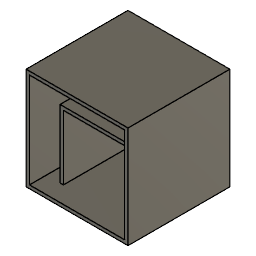
Vision globale du cube central (Autodesk Fusion 360 design; units mm, degrees)
part number: 2026-03-24-15-33-27-317
Autodesk Fusion 360 part; units mm, degrees
sketch "Esquisse1" plane through (0, 0, 0) normal (0, 0, 1) x (1, 0, 0)
  line L0 (0, 0) -> (30, 0)
  line L1 (30, 0) -> (30, 30)
  line L2 (30, 30) -> (0, 30)
  line L3 (0, 30) -> (0, 0)
  dimension "d1" = 30
  dimension "d2" = 30
  constraint horizontal L0
  constraint vertical L1
  constraint horizontal L2
  constraint vertical L3
  constraint coincident L0.start L3.end
  measures "d1" distance of L0.start L0.end
  measures "d2" distance of L0.start L2.end
extrude "Extrusion1" add sketch "Esquisse1" along normal blind 30
shell "Coque2" thickness 1 removed faces 1 at (10, 0, 10)
sketch "Esquisse5" plane through (0, 0, 1) normal (0, 0, 1) x (-1, 0, 0)
  line L0 (-1, -29) -> (-1, 0)
  line L1 (-1, 0) -> (-29, 0)
  line L2 (-29, 0) -> (-29, -29)
  line L3 (-29, -29) -> (-1, -29)
  line L4 (-5, -5) -> (-25, -5)
  line L5 (-25, -5) -> (-25, -25)
  line L6 (-25, -25) -> (-5, -25)
  line L7 (-5, -25) -> (-5, -5)
  dimension "d9" = 20
  dimension "d10" = 20
  constraint horizontal L4
  constraint vertical L5
  constraint horizontal L6
  constraint vertical L7
  measures "d9" distance of L4.start L4.end
  measures "d10" distance of L4.start L6.end
extrude "Extrusion3" add sketch "Esquisse5" along normal blind 20 contours L4 L5 L6 L7
shell "Coque3" thickness 1 removed faces 1 at (11.6667, 5, 7.6667)
